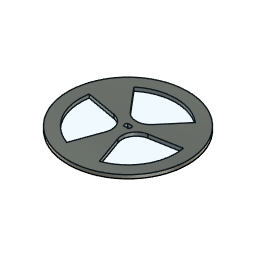
Wheel (Autodesk Fusion 360 design; units mm, degrees)
Autodesk Fusion 360 part; units mm, degrees
sketch "Sketch1" plane through (0, 0, 0) normal (0, 0, 1) x (1, 0, 0)
  circle A0 centre (0, 0) radius 50
  circle A1 centre (0, 0) radius 40
  circle A2 centre (0, 0) radius 40 construction
  line L0 (0, 40) -> (-25.7115, 30.6418) construction
  line L1 (-25.7115, 30.6418) -> (-39.3923, 6.9459) construction
  line L2 (-39.3923, 6.9459) -> (-34.641, -20) construction
  line L3 (-34.641, -20) -> (-13.6808, -37.5877) construction
  line L4 (-13.6808, -37.5877) -> (13.6808, -37.5877) construction
  line L5 (13.6808, -37.5877) -> (34.641, -20) construction
  line L6 (34.641, -20) -> (39.3923, 6.9459) construction
  line L7 (39.3923, 6.9459) -> (25.7115, 30.6418) construction
  line L8 (25.7115, 30.6418) -> (0, 40) construction
  line L9 (-13.6808, -37.5877) -> (13.6808, -37.5877) construction
  line L10 (13.6808, -37.5877) -> (34.641, -20) construction
  line L11 (34.641, -20) -> (39.3923, 6.9459) construction
  line L12 (39.3923, 6.9459) -> (25.7115, 30.6418) construction
  line L13 (25.7115, 30.6418) -> (0, 40) construction
  line L14 (-13.6808, -37.5877) -> (-34.641, -20) construction
  line L15 (-34.641, -20) -> (-39.3923, 6.9459) construction
  line L16 (-39.3923, 6.9459) -> (-25.7115, 30.6418) construction
  line L17 (-25.7115, 30.6418) -> (0, 40) construction
  line L18 (-25.7115, 30.6418) -> (-9.1649, 11.0649)
  line L19 (25.7115, 30.6418) -> (9.1649, 11.0649)
  line L20 (14.1649, 2.4046) -> (39.3923, 6.9459)
  line L21 (5, -13.4695) -> (13.6808, -37.5877)
  line L22 (-39.3923, 6.9459) -> (-14.1649, 2.4046)
  line L23 (-13.6808, -37.5877) -> (-5, -13.4695)
  arc A3 (-5, -13.4695) -> (-14.1649, 2.4046) centre (-16.2909, -9.4056) ccw
  arc A4 (14.1649, 2.4046) -> (5, -13.4695) centre (16.2909, -9.4056) ccw
  arc A5 (-9.1649, 11.0649) -> (9.1649, 11.0649) centre (0, 18.8111) ccw
  line L24 (-9.1649, 11.0649) -> (-14.1649, 2.4046) construction
  line L25 (9.1649, 11.0649) -> (14.1649, 2.4046) construction
  line L26 (-5, -13.4695) -> (5, -13.4695) construction
  line L27 (0, -37.5877) -> (0, -13.4695) construction
  line L28 (-32.5519, 18.7939) -> (-11.6649, 6.7347) construction
  line L29 (32.5519, 18.7939) -> (11.6649, 6.7347) construction
  circle A6 centre (0, 0) radius 2.62
  line L30 (-1.972, 1.725) -> (1.972, 1.725)
  line L31 (-1.972, -1.725) -> (1.972, -1.725)
  line L32 (0, 1.725) -> (0, -1.725) construction
  dimension "d1" = 100
  dimension "d2" = 10
  dimension "d8" = 12
  dimension "d9" = 12
  dimension "d10" = 12
  dimension "d11" = 10
  dimension "d15" = 5.24
  dimension "d16" = 3.45
  constraint coincident A0.centre A1.centre
  constraint concentric A0 A1
  constraint coincident A1 L0.start
  constraint coincident A1 L0.end
  constraint coincident A1 L1.end
  constraint coincident A1 L2.end
  constraint coincident A1 L3.end
  constraint coincident A1 L4.end
  constraint horizontal L4
  constraint coincident A1 L5.end
  constraint coincident A1 L6.end
  constraint coincident A1 L7.end
  constraint equal L0 L4
  constraint equal L1 L4
  constraint equal L2 L4
  constraint equal L3 L4
  constraint equal L4 L8
  constraint equal L4 L7
  constraint equal L4 L6
  constraint equal L4 L5
  constraint coincident L0 L8.end
  constraint coincident A2 L3.end
  constraint coincident A2 L4.end
  constraint horizontal L9
  constraint coincident A2 L5.end
  constraint coincident A2 L6.end
  constraint coincident A2 L7.end
  constraint coincident A2 L0.start
  constraint coincident A2 L2.end
  constraint coincident A2 L1.end
  constraint coincident A2 L0.end
  constraint equal L9 L17
  constraint equal L9 L16
  constraint equal L9 L15
  constraint equal L9 L14
  constraint equal L9 L13
  constraint equal L9 L12
  constraint equal L9 L11
  constraint equal L9 L10
  constraint coincident L0.start L8.end
  constraint coincident L1.end L22
  constraint coincident L3.end L23
  constraint tangent L22 A3
  constraint tangent L23 A3
  constraint coincident L4.end L21
  constraint coincident L6.end L20
  constraint tangent L21 A4
  constraint tangent L20 A4
  constraint coincident L0.end L18
  constraint coincident L7.end L19
  constraint tangent L18 A5
  constraint tangent L19 A5
  constraint horizontal L26
  constraint parallel L1 L24
  constraint parallel L7 L25
  constraint midpoint L4 L27.start
  constraint midpoint L26 L27.end
  constraint midpoint L1 L28.start
  constraint midpoint L24 L28.end
  constraint perpendicular L24 L28
  constraint midpoint L7 L29.start
  constraint midpoint L25 L29.end
  constraint perpendicular L25 L29
  constraint coincident A6 L30.start
  constraint coincident A6 L30.end
  constraint horizontal L30
  constraint coincident A6 L31.start
  constraint coincident A6 L31.end
  constraint parallel L30 L31
  constraint midpoint L30 L32.start
  constraint midpoint L31 L32.end
  constraint midpoint A0.centre L32
  measures "d1" diameter of A0
  measures "d2" distance of A0 A1
  measures "d8" radius of A3
  measures "d9" radius of A4
  measures "d10" radius of A5
  measures "d11" distance of L22.end L18.end
  measures "d15" diameter of A6
  measures "d16" distance of L30 L31
extrude "Extrude2" add sketch "Sketch1" along normal blind 3 contours A0 | A1 L18 L19 L20 L21 L22 L23 A3 A4 A5 | A6 L30 | A6 L31
sketch "Sketch2" plane through (0, 0, 3) normal (0, 0, 1) x (-1, 0, 0)
  arc A0 (-25.7115, -30.6418) -> (25.7115, -30.6418) centre (0, 0) ccw
  line L0 (-25.7115, -30.6418) -> (-9.1649, -11.0649)
  arc A1 (9.1649, -11.0649) -> (-9.1649, -11.0649) centre (0, -18.8111) ccw
  line L1 (9.1649, -11.0649) -> (25.7115, -30.6418)
  arc A2 (-14.1649, -2.4046) -> (-5, 13.4695) centre (-16.2909, 9.4056) ccw
  line L2 (-14.1649, -2.4046) -> (-39.3923, -6.9459)
  arc A3 (-13.6808, 37.5877) -> (-39.3923, -6.9459) centre (0, 0) ccw
  line L3 (-13.6808, 37.5877) -> (-5, 13.4695)
  arc A4 (39.3923, -6.9459) -> (13.6808, 37.5877) centre (0, 0) ccw
  line L4 (39.3923, -6.9459) -> (14.1649, -2.4046)
  arc A5 (5, 13.4695) -> (14.1649, -2.4046) centre (16.2909, 9.4056) ccw
  line L5 (5, 13.4695) -> (13.6808, 37.5877)
  arc A6 (1.972, -1.725) -> (1.972, 1.725) centre (0, 0) ccw
  line L6 (1.972, -1.725) -> (-1.972, -1.725)
  arc A7 (-1.972, 1.725) -> (-1.972, -1.725) centre (0, 0) ccw
  line L7 (-1.972, 1.725) -> (1.972, 1.725)
  circle A8 centre (0, 0) radius 50
extrude "Extrude1" [rolled back] along distance 3 taper angle 0
equation "d15 = ( 2.62 * 2 ) * 1 mm"
